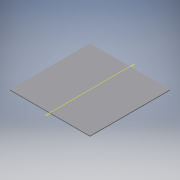
# Autodesk Inventor part: Deck
Saved by Autodesk Inventor 2018.1 (Build 221171000, 171)
## iProperties
Created: 2017-10-07
Part Number: Deck
Material: Polycarbonate, Smoke
Document SubType Name: Modeling
Designer: steele
Density: 1.2 g/cm^3
Appearance: Polycarbonate - Smoked
Mass: 3854.24 g
Surface Area: 10296.8 cm^2
Volume: 3211.86 cm^3
Author: steele
Autodesk Inventor part; units mm, degrees
ref_plane "XZ Plane" through (0, 0, 0) normal (0, 1, 0) x (-1, 0, 0)
ref_plane "XY Plane" through (0, 0, 0) normal (0, 0, 1) x (1, 0, 0)
sketch "Sketch1" plane through (0, 0, 0) normal (0, 1, 0) x (-1, 0, 0)
  line L0 (-355.6, 381) -> (-355.6, -381)
  line L1 (-355.6, -381) -> (355.6, -381)
  line L2 (355.6, -381) -> (355.6, 381)
  line L3 (355.6, 381) -> (-355.6, 381)
  line L4 (-355.6, 381) -> (355.6, -381) construction
  line L5 (-355.6, -381) -> (355.6, 381) construction
  point P0 (0, 0)
  dimension "d2" = 711.2
  dimension "d3" = 762
  constraints: 12 end point, 2 midpoint, 2 parallel, 1 perpendicular, 1 vertical
  measures "d2" distance of L0.end L1.end
  measures "d3" distance of L0.start L0.end
extrude "Extrusion1" add sketch "Sketch1" along normal blind 6.35
body "Solid1"
